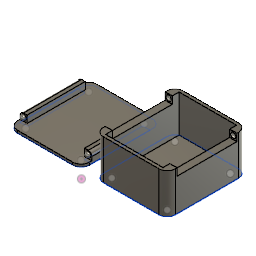
BaseBox v2 (Autodesk Fusion 360 design; units mm, degrees)
Autodesk Fusion 360 part; units mm, degrees
form "Form1" [no effect]
sketch "Bases" plane through (0, 0, 0) normal (0, 1, 0) x (1, 0, 0)
  line L0 (6.9598, 3.7095) -> (33.7098, 3.7095)
  line L1 (37.7098, 7.7095) -> (37.7098, 38.2095)
  line L2 (33.7098, 42.2095) -> (6.9598, 42.2095)
  line L3 (2.9598, 38.2095) -> (2.9598, 7.7095)
  arc A0 (6.9598, 42.2095) -> (2.9598, 38.2095) centre (6.9598, 38.2095) ccw
  arc A1 (37.7098, 38.2095) -> (33.7098, 42.2095) centre (33.7098, 38.2095) ccw
  arc A2 (33.7098, 3.7095) -> (37.7098, 7.7095) centre (33.7098, 7.7095) ccw
  arc A3 (2.9598, 7.7095) -> (6.9598, 3.7095) centre (6.9598, 7.7095) ccw
  arc A4 (2.9598, 7.7095) -> (6.9598, 3.7095) centre (6.9598, 7.7095) ccw
  arc A5 (33.7098, 3.7095) -> (37.7098, 7.7095) centre (33.7098, 7.7095) ccw
  line L4 (2.9598, 38.2095) -> (2.9598, 7.7095)
  line L5 (37.7098, 7.7095) -> (37.7098, 38.2095)
  line L6 (6.9598, 3.7095) -> (33.7098, 3.7095)
  arc A6 (6.9598, 42.2095) -> (2.9598, 38.2095) centre (6.9598, 38.2095) ccw
  line L7 (33.7098, 42.2095) -> (6.9598, 42.2095)
  arc A7 (37.7098, 38.2095) -> (33.7098, 42.2095) centre (33.7098, 38.2095) ccw
  line L8 (-38.5963, 38.1657) -> (-38.5963, 7.6657)
  arc A8 (-7.8463, 3.6657) -> (-3.8463, 7.6657) centre (-7.8463, 7.6657) ccw
  line L9 (-34.5963, 3.6657) -> (-7.8463, 3.6657)
  line L10 (-7.8463, 42.1657) -> (-34.5963, 42.1657)
  arc A9 (-34.5963, 42.1657) -> (-38.5963, 38.1657) centre (-34.5963, 38.1657) ccw
  arc A10 (-3.8463, 38.1657) -> (-7.8463, 42.1657) centre (-7.8463, 38.1657) ccw
  arc A11 (-38.5963, 7.6657) -> (-34.5963, 3.6657) centre (-34.5963, 7.6657) ccw
  line L11 (-3.8463, 7.6657) -> (-3.8463, 38.1657)
  line L12 (-38.5963, 36.9657) -> (-35.0963, 36.9657)
  line L13 (-35.0963, 36.9657) -> (-35.0963, 8.8657)
  line L14 (-35.0963, 8.8657) -> (-38.5963, 8.8657)
  line L15 (-38.5963, 8.8657) -> (-38.5963, 36.9657)
  line L16 (-3.8463, 36.9657) -> (-7.3463, 36.9657)
  line L17 (-7.3463, 36.9657) -> (-7.3463, 8.8657)
  line L18 (-7.3463, 8.8657) -> (-3.8463, 8.8657)
  line L19 (-3.8463, 8.8657) -> (-3.8463, 36.9657)
  dimension "d14" = 4
  dimension "d15" = 4
  dimension "d16" = 38.5
  dimension "d18" = 34.75
  dimension "d31" = 4
  dimension "d32" = 4
  dimension "d33" = 38.5
  dimension "d34" = 34.75
  dimension "d35" = 4
  dimension "d36" = 4
  dimension "d37" = 38.5
  dimension "d38" = 34.75
  dimension "d45" = 28.1
  dimension "d46" = 3.5
  dimension "d47" = 3.5
  measures "d14" radius of A0
  measures "d15" radius of A1
  measures "d16" distance of L0 L2
  measures "d18" distance of L1 L3
  measures "d31" radius of A6
  measures "d32" radius of A7
  measures "d33" distance of L6 L7
  measures "d34" distance of L4 L5
  measures "d35" radius of A9
  measures "d36" radius of A10
  measures "d37" distance of L9 L10
  measures "d38" distance of L8 L11
  measures "d45" distance of origin
extrude "Extrude1" add sketch "Bases" along normal blind 19.25 contours L0 L1 L2 L3 A0 A1 A2 A3 A4 A5 L4 L5 L6 A6 L7 A7 makes body 1
sketch "TopBox" plane through (0, 19.25, 0) normal (0, 1, 0) x (-1, 0, 0)
  arc A0 (-2.9598, -7.7095) -> (-6.9598, -3.7095) centre (-6.9598, -7.7095) ccw
  line L0 (-6.9598, -3.7095) -> (-33.7098, -3.7095)
  arc A1 (-33.7098, -3.7095) -> (-37.7098, -7.7095) centre (-33.7098, -7.7095) ccw
  line L1 (-37.7098, -7.7095) -> (-37.7098, -38.2095)
  arc A2 (-37.7098, -38.2095) -> (-33.7098, -42.2095) centre (-33.7098, -38.2095) ccw
  line L2 (-33.7098, -42.2095) -> (-6.9598, -42.2095)
  arc A3 (-6.9598, -42.2095) -> (-2.9598, -38.2095) centre (-6.9598, -38.2095) ccw
  line L3 (-2.9598, -38.2095) -> (-2.9598, -7.7095)
  line L4 (-6.4598, -5.2095) -> (-34.2098, -5.2095)
  line L5 (-34.2098, -5.2095) -> (-34.2098, -40.7095)
  line L6 (-34.2098, -40.7095) -> (-6.4598, -40.7095)
  line L7 (-6.4598, -40.7095) -> (-6.4598, -5.2095)
  line L8 (-2.9598, -37.4095) -> (-6.4598, -37.4095)
  line L9 (-6.4598, -37.4095) -> (-6.4598, -8.5095)
  line L10 (-6.4598, -8.5095) -> (-2.9598, -8.5095)
  line L11 (-2.9598, -8.5095) -> (-2.9598, -37.4095)
  line L12 (-34.2098, -37.4095) -> (-37.7098, -37.4095)
  line L13 (-37.7098, -37.4095) -> (-37.7098, -8.5095)
  line L14 (-37.7098, -8.5095) -> (-34.2098, -8.5095)
  line L15 (-34.2098, -8.5095) -> (-34.2098, -37.4095)
  dimension "d22" = 35.5
  dimension "d23" = 27.75
  dimension "d24" = 1.5
  dimension "d25" = 3.5
  dimension "d28" = 28.9
  measures "d24" distance of L0 L4
  measures "d25" distance of L3 L7
extrude "Extrude2" cut sketch "TopBox" against normal blind 18 contours L4 L5 L6 L7 L9 L15 bodies 1
extrude "Extrude3" cut sketch "TopBox" against normal blind 3.5 contours L3 L7 L8 L9 L10 L11 | L1 L5 L12 L13 L14 L15 bodies 1
extrude "Extrude4" add sketch "Bases" along normal blind 1.25 separate body contours L8 A8 L9 L10 A9 A10 A11 L11 L12 L13 L14 L16 L17 L18 | L8 L12 L13 L14 L15 | L11 L16 L17 L18 L19 makes body 2
extrude "Extrude5" add sketch "Bases" along normal blind 4.75 contours L8 L12 L13 L14 L15 | L11 L16 L17 L18 L19 bodies 2
fillet "Fillet1" radius 1.75 1 edges at (-3.8463, 4.75, -22.9157) on bodies 2
fillet "Fillet1" radius 1.75 1 edges at (-38.5963, 4.75, -22.9157) on bodies 2
sphere "SpherePrimitive2" cut diameter 2.5 placed x (1, 0, 0) y (0, 1, 0) z (0, 0, 1) at (35.9598, 17.5, -37.4095) bodies 1
pattern_linear "R-Pattern1" count 2 spacing 28.9 along (0, 0, 1) count 2 spacing 31.25 along (-1, 0, 0) of "SpherePrimitive2"
sphere "SpherePrimitive7" add diameter 2.5 placed x (-1, 0, 0) y (0, 1, 0) z (0, 0, -1) at (-5.5963, 3, -36.9657) bodies 2
pattern_linear "R-Pattern2" count 2 spacing 28.1 along (0, 0, 1) count 2 spacing 31.25 along (-1, 0, 0) of "SpherePrimitive7"
sketch "CutSpheres" plane through (0, 1.25, 0) normal (0, 1, 0) x (-1, 0, 0)
  line L0 (7.3463, -36.9657) -> (3.8463, -36.9657)
  line L1 (3.8463, -36.9657) -> (3.8463, -38.1657)
  arc A0 (3.8463, -38.1657) -> (7.8463, -42.1657) centre (7.8463, -38.1657) ccw
  line L2 (7.8463, -42.1657) -> (34.5963, -42.1657)
  arc A1 (34.5963, -42.1657) -> (38.5963, -38.1657) centre (34.5963, -38.1657) ccw
  line L3 (38.5963, -38.1657) -> (38.5963, -36.9657)
  line L4 (38.5963, -36.9657) -> (35.0963, -36.9657)
  line L5 (35.0963, -36.9657) -> (35.0963, -8.8657)
  line L6 (35.0963, -8.8657) -> (38.5963, -8.8657)
  line L7 (38.5963, -8.8657) -> (38.5963, -7.6657)
  arc A2 (38.5963, -7.6657) -> (34.5963, -3.6657) centre (34.5963, -7.6657) ccw
  line L8 (34.5963, -3.6657) -> (7.8463, -3.6657)
  arc A3 (7.8463, -3.6657) -> (3.8463, -7.6657) centre (7.8463, -7.6657) ccw
  line L9 (3.8463, -7.6657) -> (3.8463, -8.8657)
  line L10 (3.8463, -8.8657) -> (7.3463, -8.8657)
  line L11 (7.3463, -8.8657) -> (7.3463, -36.9657)
  line L12 (6.8463, -38.2157) -> (4.3463, -38.2157)
  line L13 (4.3463, -38.2157) -> (4.3463, -37.5157)
  line L14 (4.3463, -37.5157) -> (6.8463, -37.5157)
  line L15 (6.8463, -37.5157) -> (6.8463, -38.2157)
  line L16 (3.8463, -7.6657) -> (3.8463, -38.1657)
  line L17 (3.8463, -36.9657) -> (7.3463, -36.9657)
  line L18 (6.8463, -8.3157) -> (4.3463, -8.3157)
  line L19 (4.3463, -8.3157) -> (4.3463, -7.6157)
  line L20 (4.3463, -7.6157) -> (6.8463, -7.6157)
  line L21 (6.8463, -7.6157) -> (6.8463, -8.3157)
  line L22 (38.0963, -8.3157) -> (35.5963, -8.3157)
  line L23 (35.5963, -8.3157) -> (35.5963, -7.6157)
  line L24 (35.5963, -7.6157) -> (38.0963, -7.6157)
  line L25 (38.0963, -7.6157) -> (38.0963, -8.3157)
  line L26 (38.0963, -38.2157) -> (35.5963, -38.2157)
  line L27 (35.5963, -38.2157) -> (35.5963, -37.5157)
  line L28 (35.5963, -37.5157) -> (38.0963, -37.5157)
  line L29 (38.0963, -37.5157) -> (38.0963, -38.2157)
  line L30 (7.3463, -8.8657) -> (3.8463, -8.8657)
  line L31 (35.0963, -8.8657) -> (38.5963, -8.8657)
  line L32 (38.5963, -36.9657) -> (35.0963, -36.9657)
  line L33 (38.5963, -38.1657) -> (38.5963, -7.6657)
  dimension "d71" = 0.5
  dimension "d72" = 2.5
  dimension "d73" = 0.55
  dimension "d74" = 0.7
  dimension "d77" = 0.55
  dimension "d78" = 0.55
  dimension "d79" = 0.55
  dimension "d80" = 0.7
  dimension "d81" = 0.7
  dimension "d82" = 0.7
  dimension "d83" = 0.5
  dimension "d84" = 0.5
  dimension "d85" = 0.5
  dimension "d86" = 2.5
  dimension "d87" = 2.5
  dimension "d88" = 2.5
  measures "d71" distance of L13 L16
  measures "d73" distance of L14 L17
  measures "d77" distance of L18 L30
  measures "d78" distance of L22 L31
  measures "d79" distance of L28 L32
  measures "d83" distance of L16 L19
  measures "d84" distance of L25 L33
  measures "d85" distance of L29 L33
extrude "Extrude6" [rolled back] along distance 3 taper angle 0
equation "_width = 35.5 mm" comment "width of the box (affects the length of the hinges)"
equation "_length = 27.75 mm" comment "length of the box"
equation "_height = 18 mm" comment "height of the box"
equation "_rounding = 4 mm" comment "rounding radius of the corners of the box"
equation "_minimumWallThickness = 0.5 mm" comment "thickness of the walls around the magnets"
equation "_sidewallThickness = 1.5 mm" comment "thickness of the side walls without the hinge"
equation "_horizontalThickness = 1.25 mm" comment "thickness of the bottom of the box or the top of the lid"
equation "_magnetDiameter = 2.5 mm" comment "diameter of magnets in the hinge"
equation "_magnetHeight = 1 mm" comment "height magnets in the hinge"
equation "_hingeGap = 0.4 mm" comment "gap bewteen the lid and box parts"
equation "_hingeOverlap = 0.15 mm" comment "Size of lid's spheres that go into box holes"
equation "d14 = _rounding"
equation "d15 = _rounding"
equation "d16 = _width + 2 * _sidewallThickness"
equation "d18 = _length + 4 * _minimumWallThickness + 2 * _magnetDiameter"
equation "d20 = _height + _horizontalThickness"
equation "d22 = _width"
equation "d23 = _length"
equation "d24 = _sidewallThickness"
equation "d25 = 2 * _minimumWallThickness + _magnetDiameter"
equation "d26 = -_height"
equation "d28 = _width + 2 * _sidewallThickness - 2 * _rounding - 2 * _magnetHeight + _hingeGap"
equation "d29 = -_magnetDiameter - 2 * _minimumWallThickness"
equation "d31 = _rounding"
equation "d32 = _rounding"
equation "d33 = _width + 2 * _sidewallThickness"
equation "d34 = _length + 4 * _minimumWallThickness + 2 * _magnetDiameter"
equation "d35 = _rounding"
equation "d36 = _rounding"
equation "d37 = _width + 2 * _sidewallThickness"
equation "d38 = _length + 4 * _minimumWallThickness + 2 * _magnetDiameter"
equation "d43 = _horizontalThickness"
equation "d45 = _width + 2 * _sidewallThickness - 2 * _rounding - 2 * _magnetHeight - _hingeGap"
equation "d46 = _magnetDiameter + 2 * _minimumWallThickness"
equation "d47 = _magnetDiameter + 2 * _minimumWallThickness"
equation "d48 = _horizontalThickness + _magnetDiameter + 2 * _minimumWallThickness"
equation "d50 = ( _magnetDiameter + 2 * _minimumWallThickness ) / 2"
equation "d51 = ( _magnetDiameter + 2 * _minimumWallThickness ) / 2"
equation "d53 = _magnetDiameter"
equation "d59 = _width + 2 * _sidewallThickness - 2 * _rounding - 2 * _magnetHeight + _hingeGap"
equation "d60 = -_length - _magnetDiameter - 2 * _minimumWallThickness"
equation "d64 = _width + 2 * _sidewallThickness - 2 * _rounding - 2 * _magnetHeight - _hingeGap"
equation "d65 = -_length - _magnetDiameter - 2 * _minimumWallThickness"
equation "d71 = _minimumWallThickness"
equation "d72 = _magnetDiameter"
equation "d73 = _hingeGap + _hingeOverlap"
equation "d74 = _magnetDiameter / 2 - _hingeGap - _hingeOverlap"
equation "d75 = _minimumWallThickness + _magnetDiameter"
equation "d77 = _hingeGap + _hingeOverlap"
equation "d78 = _hingeGap + _hingeOverlap"
equation "d79 = _hingeGap + _hingeOverlap"
equation "d80 = _magnetDiameter / 2 - _hingeGap - _hingeOverlap"
equation "d81 = _magnetDiameter / 2 - _hingeGap - _hingeOverlap"
equation "d82 = _magnetDiameter / 2 - _hingeGap - _hingeOverlap"
equation "d83 = _minimumWallThickness"
equation "d84 = _minimumWallThickness"
equation "d85 = _minimumWallThickness"
equation "d86 = _magnetDiameter"
equation "d87 = _magnetDiameter"
equation "d88 = _magnetDiameter"
equation "d89 = _magnetDiameter"
